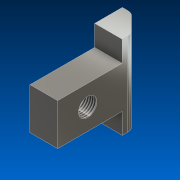
# Autodesk Inventor part: Apoio móvel da ponte
Saved by Autodesk Inventor 2016 (Build 200138000, 138)
## iProperties
Created: 2018-12-09
Part Number: Apoio móvel da ponte
Material: Generic
Document SubType Name: Modeling
Designer: lesly
Density: 1 g/cm^3
Appearance: Steel - Polished
Author: lesly
Autodesk Inventor part; units mm, degrees
ref_plane "YZ Plane" through (0, 0, 0) normal (1, 0, 0) x (0, 1, 0)
ref_plane "XZ Plane" through (0, 0, 0) normal (0, 1, 0) x (-1, 0, 0)
ref_plane "XY Plane" through (0, 0, 0) normal (0, 0, 1) x (1, 0, 0)
sketch "Sketch1" plane through (0, 0, 0) normal (1, 0, 0) x (0, 1, 0)
  line L0 (5.3982, 6.0675) -> (2.3982, 6.0675)
  line L1 (2.3982, 6.0675) -> (2.3982, -2.9325)
  line L2 (2.3982, -2.9325) -> (5.3982, -2.9325)
  line L3 (5.3982, -2.9325) -> (5.3982, 6.0675)
  point P0 (0, 0)
  dimension "d0" = 3
  dimension "d1" = 9
  constraints: 8 end point, 2 parallel, 1 horizontal, 1 perpendicular
  measures "d0" distance of L2.end L1.end
  measures "d1" distance of L1.end L0.end
extrude "Extrusion1" add sketch "Sketch1" along normal mid plane 3
sketch "Sketch2" plane through (-1.5, 2.3982, 6.0675) normal (0, 0, 1) x (1, 0, 0)
  line L0 (0, 3) -> (3, 3) projected
  line L1 (0, 3) -> (0.5858, 3)
  line L2 (3, 3) -> (3, 0) projected
  line L3 (3, 0) -> (3, 0.5858)
  line L4 (1.2929, 2.7071) -> (2.7071, 1.2929)
  arc A0 (1.2929, 2.7071) -> (0.5858, 3) centre (0.5858, 2) ccw
  arc A1 (3, 0.5858) -> (2.7071, 1.2929) centre (2, 0.5858) ccw
  line L5 (0.5858, 3) -> (3, 3)
  arc A2 (1.2929, 2.7071) -> (0.5858, 3) centre (0.5858, 2) ccw
  arc A3 (3, 0.5858) -> (2.7071, 1.2929) centre (2, 0.5858) ccw
  line L6 (3, 3) -> (3, 0.5858)
  point P0 (1.5, -2.3982)
  point P1 (1, 3)
  point P2 (3, 1)
  dimension "d5" = 1
  constraints: 10 end point, 8 point on circle, 7 point on line, 6 tangent, 4 centre point, 1 collinear, 1 concentric, 1 equal radius
  measures "d5" distance of L2.end point (3, 1)
extrude "Extrusion2" cut sketch "Sketch2" against normal blind 50
sketch "Sketch4" plane through (-1.5, 0, 0) normal (-1, 0, 0) x (0, 0, 1)
  line L0 (6.0675, 5.3982) -> (-2.9325, 5.3982) projected
  line L1 (6.0675, 2.3982) -> (-2.9325, 2.3982) projected
  line L2 (6.0675, 3.6911) -> (-2.9325, 3.6911) projected
  line L3 (1.5675, 3.6911) -> (2.5531, 5.3982)
  line L4 (1.5675, 3.6911) -> (3.5387, 3.6911) construction
  line L5 (1.5675, 3.6911) -> (0.5819, 5.3982)
  line L6 (0.5819, 5.3982) -> (2.5531, 5.3982)
  point P0 (0, 0)
  dimension "d10" = 60
  constraints: 8 end point, 2 horizontal, 1 equal length, 1 midpoint, 1 point on line
  measures "d10" angle of L4 L3
extrude "Extrusion3" cut sketch "Sketch4" against normal blind 50
sketch "Sketch5" plane through (-1.5, 2.3982, -2.9325) normal (0, -1, 0) x (1, 0, 0)
  line L0 (3, 9) -> (3, 0) projected
  line L1 (0, 0) -> (0, 9) projected
  line L2 (0, 6.75) -> (3, 6.75)
  line L3 (0, 2.25) -> (3, 2.25)
  line L4 (0, 2.25) -> (0, 6.75)
  line L5 (3, 2.25) -> (3, 6.75)
  point P0 (1.5, 2.9325)
  point P1 (0, 4.5)
  constraints: 8 end point, 2 collinear, 2 point on line, 1 horizontal
extrude "Extrusion4" add sketch "Sketch5" along normal blind 7
sketch "Sketch7" plane through (-1.5, 0, 0) normal (-1, 0, 0) x (0, 0, 1)
  line L0 (-2.9325, 2.3982) -> (-0.6825, 2.3982) projected
  circle A0 centre (1.6026, -1.3518) radius 1
  point P0 (0.6868, -0.5794)
  constraints: 1 centre point
extrude "Extrusion5" cut sketch "Sketch7" against normal blind 10
thread "Thread1" size "M2x0.25" class "6H" standard "ANSI Metric M Profile" full length
body "Solid1"
